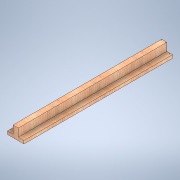
# Autodesk Inventor part: Madera
Saved by Autodesk Inventor 2020 (Build 240168000, 168)
## iProperties
Created: 2022-03-23
Part Number: Madera
Material: Madera (abedul)
Document SubType Name: Modeling
Designer: aarco
Density: 0.55 g/cm^3
Appearance: Abedul - Natural pulido
Author: aarco
Autodesk Inventor part; units mm, degrees
ref_plane "YZ Plane" through (0, 0, 0) normal (1, 0, 0) x (0, 1, 0)
ref_plane "XZ Plane" through (0, 0, 0) normal (0, 1, 0) x (-1, 0, 0)
ref_plane "XY Plane" through (0, 0, 0) normal (0, 0, 1) x (1, 0, 0)
sketch "Boceto1" plane through (0, 0, 0) normal (0, 1, 0) x (-1, 0, 0)
  line L0 (50, 450) -> (-50, 450)
  line L1 (-50, 450) -> (-50, -450)
  line L2 (-50, -450) -> (50, -450)
  line L3 (50, -450) -> (50, 450)
  line L4 (0, 450) -> (0, 0) construction
  line L5 (0, 0) -> (-50, 0) construction
  dimension "d0" = 100
  dimension "d1" = 900
  constraints: 12 end point, 3 perpendicular, 2 midpoint, 2 parallel, 1 horizontal
  measures "d0" distance of L0.start L0.end
  measures "d1" distance of L2.end L0.start
extrude "Extrusión1" add sketch "Boceto1" along normal blind 19
sketch "Boceto2" plane through (0, 19, 0) normal (0, 1, 0) x (1, 0, 0)
  line L0 (-50, -450) -> (50, -450) projected
  line L1 (-16, -450) -> (16, -450)
  line L2 (16, -450) -> (16, 450)
  line L3 (16, 450) -> (-16, 450)
  line L4 (-16, 450) -> (-16, -450)
  line L5 (50, 450) -> (-50, 450) projected
  point P0 (0, 0)
  point P1 (0, -450)
  dimension "d4" = 32
  constraints: 8 end point, 2 midpoint, 2 parallel, 2 point on line, 1 horizontal, 1 perpendicular
  measures "d4" distance of L1.end L1.start
extrude "Extrusión2" add sketch "Boceto2" along normal blind 48
sketch "Boceto3" plane through (0, 0, 0) normal (0, -1, 0) x (1, 0, 0)
  line L0 (50, 450) -> (50, -450) projected
  line L1 (50, -444.5) -> (-50, -444.5) construction
  line L2 (-50, -450) -> (-50, 450) projected
  circle A0 centre (36.5, -444.5) radius 1.5
  circle A1 centre (13.5, -444.5) radius 1.5
  line L3 (50, -450) -> (-50, -450) projected
  line L4 (50, -444.5) -> (0, -444.5) construction
  line L5 (25, -444.5) -> (25, -433.7226) construction
  line L6 (0, -444.5) -> (0, -462.9029) construction
  circle A2 centre (-36.5, -444.5) radius 1.5
  circle A3 centre (-13.5, -444.5) radius 1.5
  point P0 (0, 0)
  dimension "d7" = 3
  dimension "d8" = 5.5
  dimension "d9" = 23
  constraints: 8 end point, 4 centre point, 4 point on line, 3 symmetric about line, 2 midpoint, 1 equal radius, 1 horizontal, 1 perpendicular, 1 vertical, 2 other
  measures "d7" diameter of A0
  measures "d8" distance between parallel lines of L1 L3
  measures "d9" distance of A1.centre A0.centre
extrude "Extrusión3" cut sketch "Boceto3" against normal through all
